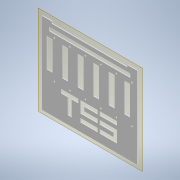
# Autodesk Inventor part: Part36
Saved by Autodesk Inventor 2020 (Build 240168000, 168)
## iProperties
Created: 2020-06-02
Part Number: Part36
Material: Generic
Document SubType Name: Sheet Metal
Designer: Gebruiker
Density: 1 g/cm^3
Sheet Metal Rule: Default_mm
Appearance: Default
Author: Gebruiker
Autodesk Inventor part; units mm, degrees
ref_plane "YZ Plane" through (0, 0, 0) normal (1, 0, 0) x (0, 1, 0)
ref_plane "XZ Plane" through (0, 0, 0) normal (0, 1, 0) x (-1, 0, 0)
ref_plane "XY Plane" through (0, 0, 0) normal (0, 0, 1) x (1, 0, 0)
ref_plane "Work Plane1" through (0, 0, 0) normal (0, 0, 1) x (1, 0, 0)
sketch "Sketch1" plane through (0, 0, 0) normal (0, 0, 1) x (1, 0, 0)
  line L0 (21.0929, -113.6856) -> (-23.9071, -113.6856)
  line L1 (-23.9071, -113.6856) -> (-23.9071, -103.6856)
  line L2 (-23.9071, -103.6856) -> (21.0929, -103.6856)
  line L3 (21.0929, -103.6856) -> (21.0929, -113.6856)
  line L4 (26.0929, -103.6856) -> (61.0929, -103.6856)
  line L5 (61.0929, -103.6856) -> (61.0929, -93.6856)
  line L6 (61.0929, -93.6856) -> (26.0929, -93.6856)
  line L7 (26.0929, -93.6856) -> (26.0929, -83.3195)
  line L8 (26.0929, -83.3195) -> (71.0929, -83.3195)
  line L9 (71.0929, -83.3195) -> (71.0929, -113.6856)
  line L10 (71.0929, -113.6856) -> (26.0929, -113.6856)
  line L11 (26.0929, -113.6856) -> (26.0929, -103.6856)
  line L12 (-13.9071, -83.6856) -> (21.0929, -83.6856)
  line L13 (21.0929, -83.6856) -> (21.0929, -93.6856)
  line L14 (21.0929, -93.6856) -> (-23.9071, -93.6856)
  line L15 (-23.9071, -93.6856) -> (-23.9071, -63.6856)
  line L16 (-23.9071, -63.6856) -> (21.0929, -63.6856)
  line L17 (21.0929, -63.6856) -> (21.0929, -73.6856)
  line L18 (21.0929, -73.6856) -> (-13.9071, -73.6856)
  line L19 (-13.9071, -73.6856) -> (-13.9071, -83.6856)
  line L20 (26.0929, -63.6856) -> (71.0929, -63.6856)
  line L21 (71.0929, -63.6856) -> (71.0929, -73.6856)
  line L22 (71.0929, -73.6856) -> (26.0929, -73.6856)
  line L23 (26.0929, -73.6856) -> (26.0929, -63.6856)
  line L24 (-28.9071, -63.6856) -> (-28.9071, -73.6856)
  line L25 (-28.9071, -73.6856) -> (-46.4071, -73.6856)
  line L26 (-46.4071, -73.6856) -> (-46.4071, -113.6856)
  line L27 (-46.4071, -113.6856) -> (-56.4071, -113.6856)
  line L28 (-56.4071, -113.6856) -> (-56.4071, -73.6856)
  line L29 (-56.4071, -73.6856) -> (-73.9071, -73.6856)
  line L30 (-73.9071, -73.6856) -> (-73.9071, -63.6856)
  line L31 (-73.9071, -63.6856) -> (-28.9071, -63.6856)
  line L32 (-103, 60.0133) -> (103, 60.0133)
  arc A0 (105, 58.0133) -> (103, 60.0133) centre (103, 58.0133) ccw
  line L33 (105, 58.0133) -> (105, 52.0133)
  arc A1 (103, 50.0133) -> (105, 52.0133) centre (103, 52.0133) ccw
  line L34 (103, 50.0133) -> (-103, 50.0133)
  arc A2 (-105, 52.0133) -> (-103, 50.0133) centre (-103, 52.0133) ccw
  line L35 (-105, 52.0133) -> (-105, 58.0133)
  arc A3 (-103, 60.0133) -> (-105, 58.0133) centre (-103, 58.0133) ccw
  line L36 (24.5, -38.5) -> (9.5, -38.5)
  line L37 (9.5, -38.5) -> (9.5, 36.5)
  line L38 (9.5, 36.5) -> (24.5, 36.5)
  line L39 (24.5, 36.5) -> (24.5, -38.5)
  line L40 (-110.5, 36.5) -> (-95.5, 36.5)
  line L41 (-95.5, 36.5) -> (-95.5, -38.5)
  line L42 (-95.5, -38.5) -> (-110.5, -38.5)
  line L43 (-110.5, -38.5) -> (-110.5, 36.5)
  line L44 (49.5, -38.5) -> (49.5, 36.5)
  line L45 (49.5, 36.5) -> (64.5, 36.5)
  line L46 (64.5, 36.5) -> (64.5, -38.5)
  line L47 (64.5, -38.5) -> (49.5, -38.5)
  line L48 (-15.5, -38.5) -> (-30.5, -38.5)
  line L49 (-30.5, -38.5) -> (-30.5, 36.5)
  line L50 (-30.5, 36.5) -> (-15.5, 36.5)
  line L51 (-15.5, 36.5) -> (-15.5, -38.5)
  line L52 (-55.5, 36.5) -> (-55.5, -38.5)
  line L53 (-55.5, -38.5) -> (-70.5, -38.5)
  line L54 (-70.5, -38.5) -> (-70.5, 36.5)
  line L55 (-70.5, 36.5) -> (-55.5, 36.5)
  line L56 (104.5, 36.5) -> (104.5, -38.5)
  line L57 (104.5, -38.5) -> (89.5, -38.5)
  line L58 (89.5, -38.5) -> (89.5, 36.5)
  line L59 (89.5, 36.5) -> (104.5, 36.5)
  circle A4 centre (29, 42) radius 2
  circle A5 centre (109, -56) radius 2
  circle A6 centre (-51, -56) radius 2
  circle A7 centre (-11, -56) radius 2
  circle A8 centre (-91, 42) radius 2
  circle A9 centre (69, 42) radius 2
  circle A10 centre (-11, 42) radius 2
  circle A11 centre (69, -56) radius 2
  circle A12 centre (-91, -56) radius 2
  circle A13 centre (29, -56) radius 2
  circle A14 centre (-51, 42) radius 2
  circle A15 centre (109, 42) radius 2
  line L60 (122.5, -135) -> (122.5, 75)
  line L61 (97.5, 75) -> (122.5, 75)
  line L62 (97.5, 70) -> (97.5, 75)
  line L63 (-97.5, 70) -> (97.5, 70)
  line L64 (-97.5, 70) -> (-97.5, 75)
  line L65 (-122.5, 75) -> (-97.5, 75)
  line L66 (-122.5, -135) -> (-122.5, 75)
  line L67 (-122.5, -135) -> (122.5, -135)
  point P0 (0, 0)
extrude "Plate1" add sketch "Sketch1" along normal blind 2
equation "\"d0\" = Thickness"
equation "\"BendRadius\" = Thickness"
equation "\"BendReliefWidth\" = Thickness"
equation "\"BendReliefDepth\" = 0.5 * Thickness"
equation "\"CornerReliefSize\" = 4 * Thickness"
equation "\"MinimumRemnant\" = 2 * Thickness"
equation "\"TransitionRadius\" = BendRadius"
equation "\"JacobiRadiusSize\" = BendRadius"
equation "\"GapSize\" = Thickness"
equation "\"Thickness\" = 2"
body "Solid1"
